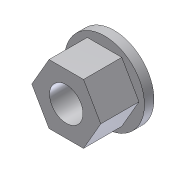
# Autodesk Inventor part: MS21042-02
Saved by Autodesk Inventor 2014 SP1 (Build 180222100, 222)
## iProperties
Created: 2012-04-24
Part Number: MS21042-02
Document SubType Name: Modeling
Designer: Robert Davis
Density: 1 g/cm^3
Description: SELF-LOCK NUT, #2-56
Material: Generic
Appearance: Default
Author: Robert Davis
Autodesk Inventor part; units mm, degrees
ref_plane "YZ Plane" through (0, 0, 0) normal (1, 0, 0) x (0, 1, 0)
ref_plane "XZ Plane" through (0, 0, 0) normal (0, 1, 0) x (-1, 0, 0)
ref_plane "XY Plane" through (0, 0, 0) normal (0, 0, 1) x (1, 0, 0)
sketch "Sketch1" plane through (0, 0, 0) normal (0, 0, 1) x (1, 0, 0)
  line L0 (0.9165, 1.5875) -> (1.8331, 0)
  line L1 (1.8331, 0) -> (0.9165, -1.5875)
  line L2 (0.9165, -1.5875) -> (-0.9165, -1.5875)
  line L3 (-0.9165, -1.5875) -> (-1.8331, 0)
  line L4 (-1.8331, 0) -> (-0.9165, 1.5875)
  line L5 (-0.9165, 1.5875) -> (0.9165, 1.5875)
  point P0 (0, 0)
  point P1 (0, 0)
  dimension "d0" = 3.175
  constraints: 12 end point, 13 other
  measures "d0" distance between parallel lines of L5 L2
extrude "Extrusion1" add sketch "Sketch1" along normal blind 2.54
sketch "Sketch2" plane through (0, 0, 0) normal (0, 0, -1) x (-1, 0, 0)
  line L0 (-0.9165, 1.5875) -> (-1.8331, 0) projected
  line L1 (-1.8331, 0) -> (-0.9165, -1.5875) projected
  line L2 (-0.9165, -1.5875) -> (0.9165, -1.5875) projected
  line L3 (0.9165, -1.5875) -> (1.8331, 0) projected
  line L4 (1.8331, 0) -> (0.9165, 1.5875) projected
  line L5 (0.9165, 1.5875) -> (-0.9165, 1.5875) projected
  circle A0 centre (0, 0) radius 2.1209
  dimension "d4" = 4.2418
  constraints: 1 centre point
  measures "d4" diameter of A0
extrude "Extrusion2" add sketch "Sketch2" against normal blind 0.508
sketch "Sketch3" plane through (0, 0, 0) normal (0, 0, -1) x (-1, 0, 0)
  circle A0 centre (0, 0) radius 0.889
  dimension "d7" = 1.778
  constraints: 1 centre point
  measures "d7" diameter of A0
extrude "Extrusion3" cut sketch "Sketch3" against normal through all
body "Solid1"
